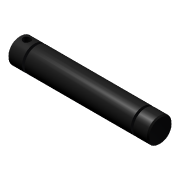
# Autodesk Inventor part: pino_a3
Saved by Autodesk Inventor 2012 SP2 (Build 160219200, 219)
## iProperties
Created: 2015-05-25
Part Number: pino_a3
Material: Aço carbono
Document SubType Name: Modeling
Designer: Projeto02
Density: 7.87 g/cm^3
Mass: 34.0168 g
Surface Area: 21.4244 cm^2
Volume: 4.32233 cm^3
Author: Projeto02
Autodesk Inventor part; units mm, degrees
ref_plane "YZ Plane" through (0, 0, 0) normal (1, 0, 0) x (0, 1, 0)
ref_plane "XZ Plane" through (0, 0, 0) normal (0, 1, 0) x (-1, 0, 0)
ref_plane "XY Plane" through (0, 0, 0) normal (0, 0, 1) x (1, 0, 0)
sketch "Esboço2" plane through (0, 0, 0) normal (1, 0, 0) x (0, 1, 0)
  circle A0 centre (0, 0) radius 5
  dimension "d0" = 10
  constraints: 1 centre point, 1 coincident
  measures "d0" diameter of A0
extrude "Extrusão1" add sketch "Esboço2" along normal blind 6
sketch "Esboço3" plane through (6, 0, 0) normal (1, 0, 0) x (0, 0, -1)
  circle A0 centre (0, 0) radius 5 projected
  circle A1 centre (0, 0) radius 3.5719
  dimension "d3" = 7.1437
  constraints: 1 centre point, 1 coincident
  measures "d3" diameter of A1
extrude "Extrusão2" add sketch "Esboço3" along normal blind 1 contours A1
sketch "Esboço4" plane through (7, 0, 0) normal (1, 0, 0) x (0, 0, -1)
  circle A0 centre (0, 0) radius 3.5719 projected
  circle A1 centre (0, 0) radius 5
  dimension "d6" = 10
  constraints: 1 centre point, 1 coincident
  measures "d6" diameter of A1
extrude "Extrusão3" add sketch "Esboço4" along normal blind 43 contours A0 | A1
sketch "Esboço8" plane through (50, 0, 0) normal (1, 0, 0) x (0, 0, -1)
  circle A0 centre (0, 0) radius 5 projected
  circle A1 centre (0, 0) radius 3.5719
  dimension "d34" = 7.1437
  constraints: 1 centre point, 1 coincident
  measures "d34" diameter of A1
extrude "Extrusão6" add sketch "Esboço8" along normal blind 1 contours A1
sketch "Esboço9" plane through (51, 0, 0) normal (1, 0, 0) x (0, 0, -1)
  circle A0 centre (0, 0) radius 3.5719 projected
  circle A1 centre (0, 0) radius 5
  dimension "d39" = 10
  constraints: 1 centre point, 1 coincident
  measures "d39" diameter of A1
extrude "Extrusão7" add sketch "Esboço9" along normal blind 6 contours A0 | A1
chamfer "Chanfro2" distance 0.5 angle 45 2 edges at (57, 0, 5) (0, -5, 0)
sketch "Esboço10" plane through (0, 0, 0) normal (0, 0, 1) x (1, 0, 0)
  line L0 (0, -4.5) -> (0, 4.5) projected
  point P0 (0, 0)
  point P1 (3, 0)
  dimension "d43" = 3
  measures "d43" distance from line of L0 point (3, 0)
hole "Furo3" at (3, 0, 0) direction (0, 0, -1) diameter 3 end through all
hole "Furo4" at (3, 0, 0) direction (0, 0, 1) diameter 3 end through all
